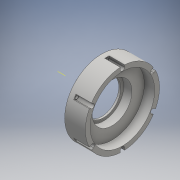
# Autodesk Inventor part: Деталь 3
Saved by Autodesk Inventor 2016 SP1 (Build 200210100, 210)
## iProperties
Created: 2016-05-02
Part Number: Деталь 3
Material: Типовые
Document SubType Name: Modeling
Designer: AS
Density: 1 g/cm^3
Appearance: По умолчанию
Author: AS
Autodesk Inventor part; units mm, degrees
ref_plane "YZ Plane" through (0, 0, 0) normal (1, 0, 0) x (0, 1, 0)
ref_plane "XZ Plane" through (0, 0, 0) normal (0, 1, 0) x (-1, 0, 0)
ref_plane "XY Plane" through (0, 0, 0) normal (0, 0, 1) x (1, 0, 0)
sketch "Эскиз1" plane through (0, 0, 0) normal (0, 0, 1) x (1, 0, 0)
  line L0 (100.7957, -43) -> (100.7957, -76)
  line L1 (100.7957, -76) -> (90.7957, -76)
  line L2 (90.7957, -76) -> (90.7957, -81)
  line L3 (90.7957, -81) -> (100.7957, -81)
  line L4 (100.7957, -81) -> (100.7957, -93)
  line L5 (100.7957, -93) -> (152.7957, -93)
  line L6 (152.7957, -93) -> (152.7957, -81)
  line L7 (152.7957, -81) -> (126.7957, -81)
  line L8 (126.7957, -81) -> (126.7957, -50)
  line L9 (126.7957, -50) -> (105.7957, -50)
  line L10 (105.7957, -50) -> (105.7957, -43)
  line L11 (105.7957, -43) -> (100.7957, -43)
  line L12 (-30.5591, 0) -> (183.3548, 0) projected
  point P0 (0, 0)
  dimension "d0" = 52
  dimension "d1" = 12
  dimension "d2" = 26
  dimension "d3" = 5
  dimension "d4" = 31
  dimension "d5" = 50
  dimension "d7" = 10
  dimension "d8" = 5
  dimension "d9" = 93
  constraints: 24 end point, 8 perpendicular, 4 point on line, 1 parallel, 1 vertical
  measures "d0" distance of L4.end L5.end
  measures "d1" distance between parallel lines of L5 L7
  measures "d2" distance of L6.end L7.end
  measures "d3" distance of L10.end L0.start
  measures "d4" distance between parallel lines of L9 L7
  measures "d5" distance between parallel lines of L11 L5
  measures "d7" distance of L0.end L1.end
  measures "d8" distance between parallel lines of L3 L1
  measures "d9" distance between parallel lines of L5 L12
revolve "Вращение1" add sketch "Эскиз1" angle 360 about axis through (-10, 0, 0) along (1, 0, 0)
chamfer "Фаска1" distance 2 angle 45 1 edges at (90.7957, 81, 0)
sketch "Эскиз2" plane through (152.7957, 0, 0) normal (1, 0, 0) x (0, 0, -1)
  arc A0 (-87.4862, -5.5) -> (-87.4862, 5.5) centre (-87.4862, 0) ccw
  line L0 (-87.4862, -5.5) -> (-100.8343, -5.5)
  line L1 (-100.8343, -5.5) -> (-100.8343, 5.5)
  line L2 (-100.8343, 5.5) -> (-87.4862, 5.5)
  point P0 (0, 0)
  dimension "d13" = 11
  constraints: 6 end point, 2 point on circle, 1 centre point, 1 horizontal, 1 perpendicular, 1 tangent
  measures "d13" diameter of A0
extrude "Выдавливание1" cut sketch "Эскиз2" against normal blind 39
pattern_circular "Круговой массив1" count 6 over 360 about axis through (-10, 0, 0) along (1, 0, 0) of "Выдавливание1"
hole "Отверстие1" at (113.7957, 0.0076, 87.3708) direction (-1, 0, 0) diameter 5 end through all counterbore diameter 9 counterbore depth 5
pattern_circular "Круговой массив2" count 6 over 360 about axis through (-10, 0, 0) along (1, 0, 0) of "Отверстие1"
